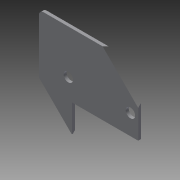
# Autodesk Inventor part: bottom pcb
Saved by Autodesk Inventor 2015 SP1 (Build 190203100, 203)
## iProperties
Created: 2015-04-28
Part Number: bottom pcb
Material: Generic
Document SubType Name: Modeling
Designer: Joseph
Density: 1 g/cm^3
Appearance: Default
Author: Joseph
Autodesk Inventor part; units mm, degrees
ref_plane "YZ Plane" through (0, 0, 0) normal (1, 0, 0) x (0, 1, 0)
ref_plane "XZ Plane" through (0, 0, 0) normal (0, 1, 0) x (-1, 0, 0)
ref_plane "XY Plane" through (0, 0, 0) normal (0, 0, 1) x (1, 0, 0)
sketch "Sketch1" plane through (0, 0, 0) normal (0, 0, 1) x (1, 0, 0)
  line L0 (5.313, -0.7489) -> (5.313, 22.2511)
  line L1 (7.313, 24.2511) -> (52.313, 24.2511)
  line L2 (54.313, 22.2511) -> (54.313, -1.4977)
  line L3 (18.7276, -1.4977) -> (18.7276, -12.4977)
  line L4 (18.7276, -12.4977) -> (5.313, -12.4977)
  line L5 (5.313, -12.4977) -> (5.313, -0.7489)
  arc A0 (7.313, 24.2511) -> (5.313, 22.2511) centre (7.313, 22.2511) ccw
  arc A1 (54.313, 22.2511) -> (52.313, 24.2511) centre (52.313, 22.2511) ccw
  line L6 (84.2832, -8.9121) -> (84.2832, 15.2621) construction
  line L7 (18.7276, -1.4977) -> (54.313, -1.4977)
  line L8 (88.3832, 16.5) -> (88.3832, -1)
  line L9 (80.1832, 16.5) -> (80.1832, -1)
  line L10 (80.1832, 3.175) -> (88.3832, 3.175) construction
  line L11 (44.5332, 6.35) -> (44.5332, -2.196) construction
  line L12 (40.0332, -2.196) -> (40.0332, 6.35) construction
  line L13 (37.5332, -2.196) -> (37.5332, 6.35) construction
  line L14 (33.0332, -2.196) -> (33.0332, 6.35) construction
  line L15 (61.1001, 16.2511) -> (10.5614, 16.2511) construction
  line L16 (-11.8823, -12.4977) -> (-2.9827, -12.4977) construction
  line L17 (-2.9827, -12.4977) -> (29.3305, -12.4977) construction
  point P0 (0, 0)
  point P1 (84.2832, 3.175)
  point P2 (13.1739, -12.4977)
  dimension "d0" = 2
  dimension "d1" = 45
  dimension "d3" = 39.75
  dimension "d5" = 4.5
  dimension "d6" = 46.75
  dimension "d7" = 4.5
  dimension "d19" = 8
  constraints: 32 end point, 6 vertical, 4 point on circle, 4 tangent, 3 midpoint, 3 point on line, 2 centre point, 2 horizontal, 2 parallel, 2 perpendicular, 1 equal radius, 4 other
  measures "d0" radius of A0
  measures "d1" distance of L1.start L1.end
  measures "d3" distance between parallel lines of L11 L6
  measures "d5" distance between parallel lines of L12 L11
  measures "d6" distance between parallel lines of L13 L6
  measures "d7" distance between parallel lines of L14 L13
  measures "d19" distance between parallel lines of L1 L15
extrude "Extrusion1" add sketch "Sketch1" along normal blind 1.2
sketch "Sketch2" plane through (0, 0, 1.2) normal (0, 0, 1) x (1, 0, 0)
  circle A0 centre (17.2003, 6.6401) radius 1.321 projected
  circle A1 centre (42.2003, 6.6401) radius 1.321 projected
  point P0 (0, 0)
  constraints: 2 coincident
hole "Hole1" at (42.2003, 6.6401, 1.2) at (17.2003, 6.6401, 1.2) direction (0, 0, -1) diameter 3.797 end through all clearance for "Flat Head Machine Screw (82)" size "#6" standard "Ansi Unified Screw Threads"
body "Solid1"
